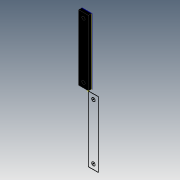
# Autodesk Inventor part: mallet_sideplate
Saved by Autodesk Inventor 2015 (Build 190159000, 159)
## iProperties
Created: 2014-08-31
Part Number: mallet_sideplate
Material: Generic
Document SubType Name: Modeling
Designer: shohei
Density: 1 g/cm^3
Appearance: Default
Mass: 58.4292 g
Surface Area: 169.142 cm^2
Volume: 58.4292 cm^3
Author: shohei
Autodesk Inventor part; units mm, degrees
ref_plane "YZ Plane" through (0, 0, 0) normal (1, 0, 0) x (0, 1, 0)
ref_plane "XZ Plane" through (0, 0, 0) normal (0, 1, 0) x (-1, 0, 0)
ref_plane "XY Plane" through (0, 0, 0) normal (0, 0, 1) x (1, 0, 0)
sketch "Block1" plane through (0, 0, 0) normal (0, 0, 1) x (1, 0, 0)
  line L0 (0.22, -200.22) -> (-30.22, -200.22)
  line L1 (-30.22, -200.22) -> (-30.22, 0.22)
  line L2 (-30.22, 0.22) -> (0.22, 0.22)
  line L3 (0.22, 0.22) -> (0.22, -200.22)
  circle A0 centre (-15, -185) radius 5.22
  circle A1 centre (-15, -15) radius 5.22
  point P0 (-15, -100)
sketch "Sketch1" plane through (0, 0, 0) normal (0, 1, 0) x (-1, 0, 0)
  line L0 (0, 0) -> (30, 0)
  line L1 (30, 0) -> (30, 200)
  line L2 (30, 200) -> (0, 200)
  line L3 (0, 200) -> (0, 0)
  circle A0 centre (15, 185) radius 5
  circle A1 centre (15, 15) radius 5
  dimension "d0" = 30
  dimension "d1" = 200
  dimension "d2" = 10
  dimension "d3" = 10
  dimension "d4" = 15
  dimension "d5" = 15
  constraints: 8 end point, 2 centre point, 2 parallel, 1 horizontal, 1 perpendicular
  measures "d0" distance of L1.end L2.end
  measures "d1" distance of L0.end L1.end
  measures "d2" diameter of A0
  measures "d3" diameter of A1
  measures "d4" distance from line of L0 A1.centre
  measures "d5" distance from line of L2 A0.centre
extrude "Extrusion1" add sketch "Sketch1" along normal blind 10
sketch "Sketch2" plane through (0, 10, 0) normal (0, 1, 0) x (1, 0, 0)
  circle A0 centre (-15, -15) radius 5 projected
  circle A1 centre (-15, -185) radius 5 projected
  line L0 (0, 0) -> (-30, 0) projected
  line L1 (-30, 0) -> (-30, -200) projected
  line L2 (-30, -200) -> (0, -200) projected
  line L3 (0, -200) -> (0, 0) projected
  constraints: 3 perpendicular, 2 other
sketch "Sketch3" plane through (0, 0, 0) normal (0, 1, 0) x (-1, 0, 0)
  point P0 (0, 0)
body "Solid1"
